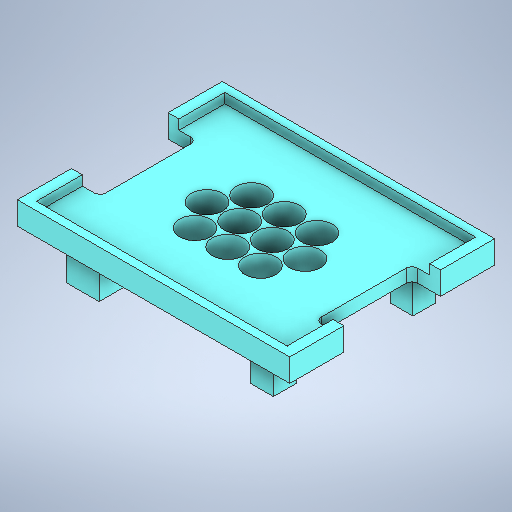
# Autodesk Inventor part: PILLARSCELLCASE18650
Saved by Autodesk Inventor 2025.2 (Build 292293000, 293)
## iProperties
Created: 2024-11-21
Part Number: PILLARSCELLCASE18650
Material: Generic
Document SubType Name: Modeling
Designer: cbast
Density: 1 g/cm^3
Appearance: Default
Mass: 190.937 g
Surface Area: 666.623 cm^2
Volume: 190.937 cm^3
Author: cbast
## iProperties of the stored document BatteryCasev1_3DPrint.ipt
Created: 2025-01-30
Part Number: BatteryCasev1_3DPrint
Material: Generic
Document SubType Name: Modeling
Designer: cbast
Density: 1 g/cm^3
Appearance: Default
Author: cbast
Autodesk Inventor part; units mm, degrees
ref_plane "YZ Plane" through (0, 0, 0) normal (1, 0, 0) x (0, 1, 0)
ref_plane "XZ Plane" through (0, 0, 0) normal (0, 1, 0) x (-1, 0, 0)
ref_plane "XY Plane" through (0, 0, 0) normal (0, 0, 1) x (1, 0, 0)
sketch "Sketch1" plane through (0, 0, 0) normal (0, 1, 0) x (-1, 0, 0)
  circle A0 centre (0, 0) radius 9.5
  circle A1 centre (20, 0) radius 9.5
  circle A2 centre (-20, 0) radius 9.5
  circle A3 centre (-10, 17.3205) radius 9.5
  circle A4 centre (10, 17.3205) radius 9.5
  circle A5 centre (30, 17.3205) radius 9.5
  circle A6 centre (10, -17.3205) radius 9.5
  circle A7 centre (30, -17.3205) radius 9.5
  circle A8 centre (-10, -17.3205) radius 9.5
  circle A9 centre (40, 0) radius 9.5
  line L0 (0, 0) -> (-32.9562, 0) construction
  line L1 (-32.9562, 0) -> (61.076, 0) construction
  circle A10 centre (0, 0) radius 10.5 construction
  circle A11 centre (-20, 0) radius 10.5 construction
  circle A12 centre (-10, -17.3205) radius 10.5 construction
  circle A13 centre (10, -17.3205) radius 10.5 construction
  circle A14 centre (30, -17.3205) radius 10.5 construction
  circle A15 centre (40, 0) radius 10.5 construction
  circle A16 centre (20, 0) radius 10.5 construction
  circle A17 centre (30, 17.3205) radius 10.5 construction
  circle A18 centre (10, 17.3205) radius 10.5 construction
  circle A19 centre (-10, 17.3205) radius 10.5 construction
  circle A20 centre (40, 0) radius 11.5 construction
  circle A21 centre (30, -17.3205) radius 11.5 construction
  circle A22 centre (10, -17.3205) radius 11.5 construction
  circle A23 centre (-10, -17.3205) radius 11.5 construction
  circle A24 centre (-20, 0) radius 11.5 construction
  circle A25 centre (-10, 17.3205) radius 11.5 construction
  circle A26 centre (10, 17.3205) radius 11.5 construction
  circle A27 centre (30, 17.3205) radius 11.5 construction
  circle A28 centre (0, 0) radius 11.5 construction
  circle A29 centre (20, 0) radius 11.5 construction
  arc A30 (39.9181, -11.4997) -> (39.9181, 11.4997) centre (39.9181, 0) ccw
  arc A31 (39.9181, 11.4997) -> (20, 22.9994) centre (30, 17.3205) ccw
  arc A32 (20, 22.9994) -> (0, 22.9994) centre (10, 17.3205) ccw
  arc A33 (0, 22.9994) -> (-19.9181, 11.4997) centre (-10, 17.3205) ccw
  arc A34 (-19.9181, 11.4997) -> (-19.9181, -11.4997) centre (-20, 0) ccw
  arc A35 (-19.9181, -11.4997) -> (0, -22.9994) centre (-10, -17.3205) ccw
  arc A36 (0, -22.9994) -> (20, -22.9994) centre (10, -17.3205) ccw
  arc A37 (20, -22.9994) -> (39.9181, -11.4997) centre (30, -17.3205) ccw
  point P0 (28.893, 7.4235)
  dimension "d0" = 19
  dimension "d2" = 19
  dimension "d4" = 19
  dimension "d6" = 19
  dimension "d8" = 19
  dimension "d10" = 19
  dimension "d11" = 19
  dimension "d13" = 19
  dimension "d14" = 19
  dimension "d53" = 19
  dimension "d91" = 1
  dimension "d144" = 21
  dimension "d145" = 21
  dimension "d146" = 21
  dimension "d147" = 21
  dimension "d148" = 21
  dimension "d149" = 21
  dimension "d150" = 21
  dimension "d151" = 21
  dimension "d152" = 21
  dimension "d153" = 21
  dimension "d154" = 23
  dimension "d155" = 23
  dimension "d156" = 23
  dimension "d157" = 23
  dimension "d158" = 23
  dimension "d159" = 23
  dimension "d160" = 23
  dimension "d161" = 23
  dimension "d162" = 23
  dimension "d163" = 23
  constraints: 38 centre point, 32 point on circle, 22 coincident, 16 tangent, 9 concentric, 4 end point, 2 point on line, 1 horizontal
  measures "d0" diameter of A0
  measures "d2" diameter of A1
  measures "d4" diameter of A2
  measures "d6" diameter of A3
  measures "d8" diameter of A4
  measures "d10" diameter of A5
  measures "d11" diameter of A6
  measures "d13" diameter of A7
  measures "d14" diameter of A8
  measures "d53" diameter of A9
  measures "d144" diameter of A10
  measures "d145" diameter of A11
  measures "d146" diameter of A12
  measures "d147" diameter of A13
  measures "d148" diameter of A14
  measures "d149" diameter of A15
  measures "d150" diameter of A16
  measures "d151" diameter of A17
  measures "d152" diameter of A18
  measures "d153" diameter of A19
  measures "d154" diameter of A20
  measures "d155" diameter of A21
  measures "d156" diameter of A22
  measures "d157" diameter of A23
  measures "d158" diameter of A24
  measures "d159" diameter of A25
  measures "d160" diameter of A26
  measures "d161" diameter of A27
  measures "d162" diameter of A28
  measures "d163" diameter of A29
extrude "Extrusion1" add sketch "Sketch1" along normal blind 15
sketch "Sketch4" plane through (0, 15, 0) normal (0, 1, 0) x (1, 0, 0)
  circle A0 centre (-30, 17.3205) radius 9.5 projected
  circle A1 centre (-40, 0) radius 9.5 projected
  circle A2 centre (-40, 0) radius 9.5 projected
  circle A3 centre (10, 17.3205) radius 9.5 projected
  circle A4 centre (-30, 17.3205) radius 9.5 projected
  circle A5 centre (-10, 17.3205) radius 9.5 projected
  circle A6 centre (-30, -17.3205) radius 9.5 projected
  circle A7 centre (-10, -17.3205) radius 9.5 projected
  circle A8 centre (10, -17.3205) radius 9.5 projected
  circle A9 centre (20, 0) radius 9.5 projected
  circle A10 centre (-20, 0) radius 9.5 projected
  circle A11 centre (0, 0) radius 9.5 projected
  line L0 (0, 0) -> (-10, 0) construction
  line L1 (-86.7, 57.7) -> (66.7, 57.7)
  line L2 (66.7, 57.7) -> (66.7, -57.7)
  line L3 (66.7, -57.7) -> (-86.7, -57.7)
  line L4 (-86.7, -57.7) -> (-86.7, 57.7)
  line L5 (-86.7, 57.7) -> (66.7, -57.7) construction
  line L6 (66.7, 57.7) -> (-86.7, -57.7) construction
  arc A12 (0, 22.9994) -> (-20, 22.9994) centre (-10, 17.3205) ccw projected
  arc A13 (19.9181, 11.4997) -> (0, 22.9994) centre (10, 17.3205) ccw projected
  arc A14 (19.9181, -11.4997) -> (19.9181, 11.4997) centre (20, 0) ccw projected
  arc A15 (0, -22.9994) -> (19.9181, -11.4997) centre (10, -17.3205) ccw projected
  arc A16 (-20, -22.9994) -> (0, -22.9994) centre (-10, -17.3205) ccw projected
  arc A17 (-39.9181, -11.4997) -> (-20, -22.9994) centre (-30, -17.3205) ccw projected
  circle A18 centre (-30, 17.3205) radius 11.5 construction
  arc A19 (-39.9181, 11.4997) -> (-39.9181, -11.4997) centre (-39.9181, 0) ccw projected
  arc A20 (-20, 22.9994) -> (-39.9181, 11.4997) centre (-30, 17.3205) ccw projected
  arc A21 (0, 22.9994) -> (-20, 22.9994) centre (-10, 17.3205) ccw
  arc A22 (19.9181, 11.4997) -> (0, 22.9994) centre (10, 17.3205) ccw
  arc A23 (19.9181, -11.4997) -> (19.9181, 11.4997) centre (20, 0) ccw
  arc A24 (0, -22.9994) -> (19.9181, -11.4997) centre (10, -17.3205) ccw
  arc A25 (-20, -22.9994) -> (0, -22.9994) centre (-10, -17.3205) ccw
  arc A26 (-39.9181, -11.4997) -> (-20, -22.9994) centre (-30, -17.3205) ccw
  arc A27 (-39.9181, 11.4997) -> (-39.9181, -11.4997) centre (-39.9181, 0) ccw
  arc A28 (-20, 22.9994) -> (-39.9181, 11.4997) centre (-30, 17.3205) ccw
  line L7 (-10.5, 0) -> (-9.5, 0) construction
  point P0 (-17.0502, -21.4927)
  point P1 (-17.0502, -11.5134)
  point P2 (-17.0502, -8.8009)
  point P3 (-17.0502, 8.8009)
  point P4 (-17.0502, 11.5134)
  point P5 (-17.0502, 21.4927)
  point P6 (-2.0059, 21.4927)
  point P7 (-2.0059, -11.5134)
  point P8 (-2.0059, -8.8009)
  point P9 (-2.0059, 8.8009)
  point P10 (-2.0059, 11.5134)
  point P11 (-2.0059, -21.4927)
  point P12 (-86.7, 0)
  point P13 (66.7, 0)
  dimension "d104" = 153.4
  dimension "d164" = 115.4
  dimension "d233" = 76.7
  dimension "d234" = 76.7
  constraints: 16 end point, 16 point on circle, 8 centre point, 8 concentric, 5 midpoint, 2 horizontal, 2 parallel, 1 perpendicular, 1 point on line, 4 other
  measures "d104" distance of L2.end L3.end
  measures "d164" distance of L1.end L2.end
  measures "d233" distance of point (-86.7, 0) L0.end
  measures "d234" distance of point (66.7, 0) L0.end
extrude "Extrusion7" add sketch "Sketch4" against normal blind 8 contours L1 L2 L3 L4
sketch "Sketch5" plane through (0, 15, 0) normal (0, 1, 0) x (1, 0, 0)
  line L0 (-86.7, -57.7) -> (66.7, -57.7) projected
  line L1 (66.7, -57.7) -> (66.7, 57.7) projected
  line L2 (66.7, 57.7) -> (-86.7, 57.7) projected
  line L3 (-86.7, 57.7) -> (-86.7, -57.7) projected
  circle A0 centre (-40, 0) radius 9.5 projected
  circle A1 centre (10, 17.3205) radius 9.5 projected
  circle A2 centre (-30, 17.3205) radius 9.5 projected
  circle A3 centre (-10, 17.3205) radius 9.5 projected
  circle A4 centre (-30, -17.3205) radius 9.5 projected
  circle A5 centre (-10, -17.3205) radius 9.5 projected
  circle A6 centre (10, -17.3205) radius 9.5 projected
  circle A7 centre (20, 0) radius 9.5 projected
  circle A8 centre (-20, 0) radius 9.5 projected
  circle A9 centre (0, 0) radius 9.5 projected
  line L4 (-86.7, 57.7) -> (66.7, 57.7)
  line L5 (66.7, 57.7) -> (66.7, -57.7)
  line L6 (66.7, -57.7) -> (-86.7, -57.7)
  line L7 (-86.7, -57.7) -> (-86.7, 57.7)
  line L8 (-93.3464, -62.7) -> (73.3464, -62.7)
  line L9 (73.3464, -62.7) -> (73.3464, 62.7)
  line L10 (73.3464, 62.7) -> (-93.3464, 62.7)
  line L11 (-93.3464, 62.7) -> (-93.3464, -62.7)
  line L12 (-93.3464, -62.7) -> (73.3464, 62.7) construction
  line L13 (73.3464, -62.7) -> (-93.3464, 62.7) construction
  point P0 (66.922, -57.45)
  point P1 (-10, 0)
  dimension "d169" = 5
  dimension "d170" = 6.6464
  dimension "d171" = 166.6929
  dimension "d172" = 125.4
  dimension "d221" = 6.6464
  constraints: 20 end point, 4 parallel, 4 point on line, 2 horizontal, 2 midpoint, 2 perpendicular
  measures "d169" distance between parallel lines of L10 L4
  measures "d170" distance between parallel lines of L9 L5
  measures "d171" distance of L9.end L10.end
  measures "d172" distance of L10.end L8.start
  measures "d221" distance between parallel lines of L3 L11
extrude "Extrusion8" add sketch "Sketch5" along normal blind 6 and the other way blind 8 contours L11 L10 L9 L8
sketch "Sketch6" plane through (0, 15, 0) normal (0, 1, 0) x (1, 0, 0)
  line L0 (59.472, 57.1514) -> (59.472, 25.95) construction
  line L1 (59.472, 25.95) -> (66.7, 25.95) construction
  line L2 (-79.472, -57.7) -> (-79.472, -25.95) construction
  line L3 (-79.472, -25.95) -> (-86.7, -25.95) construction
  circle A0 centre (59.472, 25.95) radius 3.615
  circle A1 centre (59.472, -25.95) radius 3.615
  circle A2 centre (-79.472, -25.95) radius 3.615
  circle A3 centre (-79.472, 25.95) radius 3.615
  line L4 (73.3464, -62.7) -> (73.3464, 62.7) projected
  line L5 (73.3464, 62.7) -> (-93.3464, 62.7) projected
  line L6 (-93.3464, 62.7) -> (-93.3464, -62.7) projected
  line L7 (-93.3464, -62.7) -> (73.3464, -62.7) projected
  line L8 (-86.7, -57.7) -> (-86.7, 57.7) projected
  line L9 (-86.7, 57.7) -> (66.7, 57.7) projected
  line L10 (66.7, 57.7) -> (66.7, -57.7) projected
  line L11 (66.7, -57.7) -> (-86.7, -57.7) projected
  line L12 (-86.7, -57.7) -> (66.7, -57.7) projected
  line L13 (66.7, -57.7) -> (66.7, 57.7) projected
  line L14 (66.7, 57.7) -> (-86.7, 57.7) projected
  line L15 (-86.7, 57.7) -> (-86.7, -57.7) projected
  circle A4 centre (-40, 0) radius 9.5 projected
  circle A5 centre (10, 17.3205) radius 9.5 projected
  circle A6 centre (-30, 17.3205) radius 9.5 projected
  circle A7 centre (-10, 17.3205) radius 9.5 projected
  circle A8 centre (-30, -17.3205) radius 9.5 projected
  circle A9 centre (-10, -17.3205) radius 9.5 projected
  circle A10 centre (10, -17.3205) radius 9.5 projected
  circle A11 centre (20, 0) radius 9.5 projected
  circle A12 centre (-20, 0) radius 9.5 projected
  circle A13 centre (0, 0) radius 9.5 projected
  line L16 (-86.7, 57.7) -> (66.7, 57.7)
  line L17 (66.7, 57.7) -> (66.7, -57.7)
  line L18 (66.7, -57.7) -> (-86.7, -57.7)
  line L19 (-86.7, -57.7) -> (-86.7, 57.7)
  dimension "d123" = 7.23
  dimension "d124" = 7.23
  dimension "d125" = 7.23
  dimension "d140" = 7.23
  dimension "d179" = 31.75
  dimension "d180" = 7.228
  dimension "d181" = 7.228
  dimension "d182" = 31.75
  dimension "d183" = 31.75
  dimension "d184" = 7.228
  dimension "d185" = 7.228
  dimension "d186" = 31.75
  constraints: 16 end point, 4 centre point, 2 coincident, 2 parallel, 1 horizontal, 1 perpendicular
  measures "d123" diameter of A0
  measures "d124" diameter of A1
  measures "d125" diameter of A2
  measures "d140" diameter of A3
  measures "d179" distance from line of A3.centre L16
  measures "d180" distance from line of A3.centre L15
  measures "d181" distance from line of A2.centre L8
  measures "d182" distance from line of L2.end L18
  measures "d183" distance from line of L12 A1.centre
  measures "d184" distance from line of L17 A1.centre
  measures "d185" distance from line of L17 L0.end
  measures "d186" distance from line of L16 L0.end
extrude "Extrusion6" cut sketch "Sketch6" against normal through all contours A0 | A1 | A2 | A3
sketch "Sketch7" plane through (-93.3464, 7, 62.7) normal (-1, 0, 0) x (0, 0, 1)
  line L0 (-120.4, 8) -> (-5, 8) projected
  line L1 (0, 0) -> (-125.4, 0) projected
  line L2 (-125.4, 14) -> (0, 14) projected
  line L3 (-92.265, 8) -> (-85.035, 8) projected
  line L4 (-40.365, 8) -> (-33.135, 8) projected
  line L5 (-92.265, 8) -> (-33.135, 8)
  line L6 (-33.135, 8) -> (-33.135, 14)
  line L7 (-33.135, 14) -> (-92.265, 14)
  line L8 (-92.265, 14) -> (-92.265, 8)
  point P0 (-62.7, -7)
  constraints: 8 end point, 2 parallel, 1 horizontal, 1 perpendicular, 1 point on line
extrude "Extrusion9" cut sketch "Sketch7" against normal through all
sketch "Sketch10" plane through (0, 7, 0) normal (0, -1, 0) x (1, 0, 0)
  circle A0 centre (-79.472, 25.95) radius 3.615 projected
  circle A1 centre (59.472, 25.95) radius 3.615 projected
  circle A2 centre (-79.472, -25.95) radius 3.615 projected
  circle A3 centre (59.472, -25.95) radius 3.615 projected
  line L0 (73.3464, -62.7) -> (73.3464, 62.7) projected
  line L1 (73.3464, 62.7) -> (-93.3464, 62.7) projected
  line L2 (-93.3464, 62.7) -> (-93.3464, -62.7) projected
  line L3 (-93.3464, -62.7) -> (73.3464, -62.7) projected
  arc A4 (-39.9181, -11.4997) -> (-20, -22.9994) centre (-30, -17.3205) ccw projected
  arc A5 (-39.9181, 11.4997) -> (-39.9181, -11.4997) centre (-39.9181, 0) ccw projected
  arc A6 (-20, 22.9994) -> (-39.9181, 11.4997) centre (-30, 17.3205) ccw projected
  arc A7 (0, 22.9994) -> (-20, 22.9994) centre (-10, 17.3205) ccw projected
  arc A8 (19.9181, 11.4997) -> (0, 22.9994) centre (10, 17.3205) ccw projected
  arc A9 (19.9181, -11.4997) -> (19.9181, 11.4997) centre (20, 0) ccw projected
  arc A10 (0, -22.9994) -> (19.9181, -11.4997) centre (10, -17.3205) ccw projected
  arc A11 (-20, -22.9994) -> (0, -22.9994) centre (-10, -17.3205) ccw projected
  line L4 (-93.3464, 62.7) -> (-63.3464, 62.7) construction
  line L5 (-93.3464, 62.7) -> (-93.3464, 42.7) construction
  line L6 (-93.3464, 42.7) -> (-63.3464, 42.7) construction
  line L7 (-73.3464, 52.7) -> (-53.3464, 52.7)
  line L8 (-53.3464, 52.7) -> (-53.3464, 32.7)
  line L9 (-53.3464, 32.7) -> (-73.3464, 32.7)
  line L10 (-73.3464, 32.7) -> (-73.3464, 52.7)
  line L11 (-73.3464, 52.7) -> (-53.3464, 32.7) construction
  line L12 (-53.3464, 52.7) -> (-73.3464, 32.7) construction
  line L13 (-70.8464, 50.2) -> (-55.8464, 50.2)
  line L14 (-55.8464, 50.2) -> (-55.8464, 35.2)
  line L15 (-55.8464, 35.2) -> (-70.8464, 35.2)
  line L16 (-70.8464, 35.2) -> (-70.8464, 50.2)
  line L17 (-70.8464, 50.2) -> (-55.8464, 35.2) construction
  line L18 (-55.8464, 50.2) -> (-70.8464, 35.2) construction
  line L19 (-93.3464, 0) -> (73.3464, 0) construction
  line L20 (-73.3464, -52.7) -> (-53.3464, -52.7)
  line L21 (-53.3464, -52.7) -> (-53.3464, -32.7)
  line L22 (-53.3464, -32.7) -> (-73.3464, -32.7)
  line L23 (-73.3464, -32.7) -> (-73.3464, -52.7)
  line L24 (-73.3464, -52.7) -> (-53.3464, -32.7) construction
  line L25 (-53.3464, -52.7) -> (-73.3464, -32.7) construction
  line L26 (-70.8464, -50.2) -> (-55.8464, -50.2)
  line L27 (-55.8464, -50.2) -> (-55.8464, -35.2)
  line L28 (-55.8464, -35.2) -> (-70.8464, -35.2)
  line L29 (-70.8464, -35.2) -> (-70.8464, -50.2)
  line L30 (-70.8464, -50.2) -> (-55.8464, -35.2) construction
  line L31 (-55.8464, -50.2) -> (-70.8464, -35.2) construction
  line L32 (73.3464, 62.7) -> (43.3464, 62.7) construction
  line L33 (43.3464, 62.7) -> (43.3464, 42.7) construction
  line L34 (36.3464, 49.7) -> (50.3464, 49.7)
  line L35 (50.3464, 49.7) -> (50.3464, 35.7)
  line L36 (50.3464, 35.7) -> (36.3464, 35.7)
  line L37 (36.3464, 35.7) -> (36.3464, 49.7)
  line L38 (36.3464, 49.7) -> (50.3464, 35.7) construction
  line L39 (50.3464, 49.7) -> (36.3464, 35.7) construction
  line L40 (36.3464, -49.7) -> (50.3464, -49.7)
  line L41 (50.3464, -49.7) -> (50.3464, -35.7)
  line L42 (50.3464, -35.7) -> (36.3464, -35.7)
  line L43 (36.3464, -35.7) -> (36.3464, -49.7)
  line L44 (36.3464, -49.7) -> (50.3464, -35.7) construction
  line L45 (50.3464, -49.7) -> (36.3464, -35.7) construction
  line L46 (43.3464, -42.7) -> (43.3464, -62.7) construction
  line L47 (43.3464, -42.7) -> (73.3464, -42.7) construction
  line L48 (-63.3464, -42.7) -> (-63.3464, -62.7) construction
  line L49 (-63.3464, -42.7) -> (-93.3464, -42.7) construction
  point P0 (0, 0)
  dimension "d209" = 30
  dimension "d210" = 20
  dimension "d211" = 20
  dimension "d212" = 20
  dimension "d213" = 15
  dimension "d214" = 15
  dimension "d215" = 30
  dimension "d216" = 20
  dimension "d217" = 14
  dimension "d218" = 14
  dimension "d224" = 30
  dimension "d225" = 30
  dimension "d226" = 20
  dimension "d227" = 20
  constraints: 92 end point, 14 symmetric about line, 8 midpoint, 8 point on line, 7 parallel, 6 perpendicular, 4 horizontal
  measures "d209" distance of L1.end L4.end
  measures "d210" distance of L1.end L5.end
  measures "d211" distance of L8.end L9.end
  measures "d212" distance of L7.end L8.end
  measures "d213" distance of L14.end L15.end
  measures "d214" distance of L13.end L14.end
  measures "d215" distance of L0.end L32.end
  measures "d216" distance of L32.end L33.end
  measures "d217" distance of L35.end L36.end
  measures "d218" distance of L34.end L35.end
  measures "d224" distance of L48.start L49.end
  measures "d225" distance of L46.start L47.end
  measures "d226" distance of L46.start L46.end
  measures "d227" distance of L48.start L48.end
extrude "Extrusion11" add sketch "Sketch10" along normal blind 25 contours L7 L8 L9 L10 | L23 L22 L21 L20 | L34 L35 L36 L37 | L43 L42 L41 L40
sketch "Sketch11" plane through (0, 7, 0) normal (0, -1, 0) x (1, 0, 0)
  line L0 (-70.8464, 50.2) -> (-70.8464, 35.2) projected
  line L1 (-70.8464, 35.2) -> (-55.8464, 35.2) projected
  line L2 (-55.8464, 35.2) -> (-55.8464, 50.2) projected
  line L3 (-55.8464, 50.2) -> (-70.8464, 50.2) projected
  line L4 (-70.8464, 50.2) -> (-55.8464, 50.2)
  line L5 (-55.8464, 50.2) -> (-55.8464, 35.2)
  line L6 (-55.8464, 35.2) -> (-70.8464, 35.2)
  line L7 (-70.8464, 35.2) -> (-70.8464, 50.2)
  line L8 (-55.8464, -35.2) -> (-70.8464, -35.2) projected
  line L9 (-70.8464, -35.2) -> (-70.8464, -50.2) projected
  line L10 (-70.8464, -50.2) -> (-55.8464, -50.2) projected
  line L11 (-55.8464, -50.2) -> (-55.8464, -35.2) projected
  line L12 (-70.8464, -35.2) -> (-55.8464, -35.2)
  line L13 (-55.8464, -35.2) -> (-55.8464, -50.2)
  line L14 (-55.8464, -50.2) -> (-70.8464, -50.2)
  line L15 (-70.8464, -50.2) -> (-70.8464, -35.2)
  point P0 (0, 0)
  constraints: 16 end point, 4 parallel, 2 horizontal, 2 perpendicular
extrude "Extrusion12" add sketch "Sketch11" along normal up to surface (12.5 mm away)
sketch "Sketch13" plane through (0, 7, 0) normal (0, -1, 0) x (1, 0, 0)
  line L0 (36.3464, 35.7) -> (36.3464, 49.7) projected
  line L1 (36.3464, 49.7) -> (50.3464, 49.7) projected
  line L2 (50.3464, 49.7) -> (50.3464, 35.7) projected
  line L3 (50.3464, 35.7) -> (36.3464, 35.7) projected
  line L4 (-73.3464, -32.7) -> (-53.3464, -32.7) projected
  line L5 (-53.3464, -32.7) -> (-53.3464, -52.7) projected
  line L6 (-53.3464, -52.7) -> (-73.3464, -52.7) projected
  line L7 (-73.3464, -52.7) -> (-73.3464, -32.7) projected
  line L8 (36.3464, -49.7) -> (36.3464, -35.7) projected
  line L9 (36.3464, -35.7) -> (50.3464, -35.7) projected
  line L10 (50.3464, -35.7) -> (50.3464, -49.7) projected
  line L11 (50.3464, -49.7) -> (36.3464, -49.7) projected
  line L12 (-73.3464, 32.7) -> (-73.3464, 52.7) projected
  line L13 (-73.3464, 52.7) -> (-53.3464, 52.7) projected
  line L14 (-53.3464, 52.7) -> (-53.3464, 32.7) projected
  line L15 (-53.3464, 32.7) -> (-73.3464, 32.7) projected
  circle A0 centre (-79.472, 25.95) radius 3.615 projected
  circle A1 centre (59.472, 25.95) radius 3.615 projected
  circle A2 centre (-79.472, -25.95) radius 3.615 projected
  circle A3 centre (59.472, -25.95) radius 3.615 projected
  line L16 (73.3464, -62.7) -> (73.3464, 62.7) projected
  line L17 (73.3464, 62.7) -> (-93.3464, 62.7) projected
  line L18 (-93.3464, 62.7) -> (-93.3464, -62.7) projected
  line L19 (-93.3464, -62.7) -> (73.3464, -62.7) projected
  arc A4 (-39.9181, -11.4997) -> (-20, -22.9994) centre (-30, -17.3205) ccw projected
  arc A5 (-39.9181, 11.4997) -> (-39.9181, -11.4997) centre (-39.9181, 0) ccw projected
  arc A6 (-20, 22.9994) -> (-39.9181, 11.4997) centre (-30, 17.3205) ccw projected
  arc A7 (0, 22.9994) -> (-20, 22.9994) centre (-10, 17.3205) ccw projected
  arc A8 (19.9181, 11.4997) -> (0, 22.9994) centre (10, 17.3205) ccw projected
  arc A9 (19.9181, -11.4997) -> (19.9181, 11.4997) centre (20, 0) ccw projected
  arc A10 (0, -22.9994) -> (19.9181, -11.4997) centre (10, -17.3205) ccw projected
  arc A11 (-20, -22.9994) -> (0, -22.9994) centre (-10, -17.3205) ccw projected
  line L20 (-93.3464, 29.565) -> (-75.857, 29.565)
  line L21 (-75.857, 29.565) -> (-75.857, -29.565)
  line L22 (-75.857, -29.565) -> (-93.3464, -29.565)
  line L23 (-93.3464, -29.565) -> (-93.3464, 29.565)
  line L24 (-10, 27.2798) -> (-10, -25.95) construction
  line L25 (73.3464, 29.565) -> (55.857, 29.565)
  line L26 (55.857, 29.565) -> (55.857, -29.565)
  line L27 (55.857, -29.565) -> (73.3464, -29.565)
  circle A12 centre (-79.472, -25.95) radius 3.615 projected
  line L28 (-86.7, 29.565) -> (-86.7, 57.7) projected
  line L29 (-86.7, 57.7) -> (66.7, 57.7) projected
  line L30 (66.7, 57.7) -> (66.7, 29.565) projected
  line L31 (66.7, 29.565) -> (73.3464, 29.565) projected
  line L32 (73.3464, -29.565) -> (73.3464, 29.565) projected
  line L33 (66.7, -29.565) -> (73.3464, -29.565) projected
  line L34 (66.7, -29.565) -> (66.7, -57.7) projected
  line L35 (66.7, -57.7) -> (-86.7, -57.7) projected
  line L36 (-86.7, -57.7) -> (-86.7, -29.565) projected
  line L37 (-93.3464, -29.565) -> (-86.7, -29.565) projected
  line L38 (-93.3464, 29.565) -> (-93.3464, -29.565) projected
  line L39 (-93.3464, 29.565) -> (-86.7, 29.565) projected
  circle A13 centre (59.472, -25.95) radius 3.615 projected
  circle A14 centre (-79.472, 25.95) radius 3.615 projected
  circle A15 centre (-40, 0) radius 9.5 projected
  circle A16 centre (10, -17.3205) radius 9.5 projected
  circle A17 centre (-30, -17.3205) radius 9.5 projected
  circle A18 centre (-10, -17.3205) radius 9.5 projected
  circle A19 centre (-30, 17.3205) radius 9.5 projected
  circle A20 centre (-10, 17.3205) radius 9.5 projected
  circle A21 centre (10, 17.3205) radius 9.5 projected
  circle A22 centre (20, 0) radius 9.5 projected
  circle A23 centre (-20, 0) radius 9.5 projected
  circle A24 centre (0, 0) radius 9.5 projected
  circle A25 centre (59.472, 25.95) radius 3.615 projected
  line L40 (-10.5, 0) -> (-9.5, 0) construction
  point P0 (59.472, -29.565)
  point P1 (59.472, 29.565)
  point P2 (55.857, 25.95)
  point P3 (55.857, -25.95)
  point P4 (-79.472, -29.565)
  point P5 (-75.857, -25.95)
  point P6 (-75.857, 25.95)
  point P7 (-79.472, 29.565)
  dimension "d235" = 17.4895
  dimension "d236" = 17.4895
  constraints: 18 end point, 4 symmetric about line, 2 horizontal, 2 horizontal alignment, 2 parallel, 1 perpendicular, 1 point on line, 1 vertical, 2 other
  measures "d235" distance between parallel lines of L21 L18
  measures "d236" distance between parallel lines of L16 L26
extrude "Extrusion14" cut sketch "Sketch13" against normal blind 10 contours L21 A2 L22 L18 L20 A0 | L25 L16 L27 A3 L26 A1
body "Solid1"
